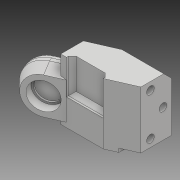
# Autodesk Inventor part: thumb_03 CMC top hinge
Saved by Autodesk Inventor 2017 SP1 (Build 210196100, 196)
## iProperties
Created: 2018-02-02
Part Number: thumb_03 CMC top hinge
Material: Generic
Document SubType Name: Modeling
Designer: JT
Density: 1 g/cm^3
Appearance: Default
Author: JT
Autodesk Inventor part; units mm, degrees
ref_plane "YZ Plane" through (0, 0, 0) normal (1, 0, 0) x (0, 1, 0)
sketch "Sketch1" plane through (0, 0, 0) normal (0, 0, 1) x (1, 0, 0)
  line L0 (0, 0) -> (-18, 0) construction
  line L1 (-9.705, 0) -> (-20.7027, -4.8012) construction
  line L2 (-20.7027, -4.8012) -> (-21.1028, -3.8847) construction
  dimension "d0" = 18
  dimension "d1" = 9.705
  dimension "d2" = 23.584
  dimension "d3" = 1
  dimension "d4" = 12
  constraints: 6 end point, 1 horizontal, 1 perpendicular, 1 point on line
  measures "d0" distance of L0.start L0.end
  measures "d1" distance of L0.start L1.start
  measures "d2" angle of L0 L1
  measures "d3" distance of L1.end L2.end
  measures "d4" distance of L1.start L1.end
ref_plane "Work Plane1" through (-20.7027, -4.8012, 0) normal (-0.4001, 0.9165, 0) x (-0.9165, -0.4001, 0)
sketch "Sketch3" plane through (-20.7027, -4.8012, 0) normal (-0.4001, 0.9165, 0) x (-0.9165, -0.4001, 0)
  circle A0 centre (0, 0) radius 6
  line L0 (0, -6) -> (-8, -6)
  line L1 (-8, -6) -> (-8, 6)
  line L2 (-8, 6) -> (0, 6)
  line L3 (0, 6) -> (0, -6)
  point P0 (-20.8944, 0)
  point P1 (0, 0)
  dimension "d8" = 12
  dimension "d13" = 8
  constraints: 8 end point, 3 horizontal, 2 parallel, 1 coincident, 1 perpendicular, 1 vertical alignment, 2 other
  measures "d13" distance from line of point (0, 0) L1
extrude "Extrusion2" add sketch "Sketch3" along normal blind 6
chamfer "Chamfer2" distance 3 angle 22 3 edges at (-26.2015, -7.2018, 0) (-17.0368, -3.2008, -6) (-17.0368, -3.2008, 6) measured on face at (-26.265, -5.0472, -3) measured on face at (-16.615, -0.8344, 6) measured on face at (-19.0589, -1.9013, -6)
sketch "Sketch2" plane through (0, 0, 0) normal (0, 0, 1) x (1, 0, 0)
  line L0 (-6.8718, -3) -> (-18, -3)
  line L1 (-18, -3) -> (-18, 2.9255)
  line L2 (-18, 2.9255) -> (0, 10.7837)
  line L3 (0, 10.7837) -> (0, 0)
  line L4 (-9.705, 0) -> (-20.7027, -4.8012) construction
  line L5 (-6.8718, -3) -> (0, 0)
  point P0 (0, 0)
  point P1 (-18, 0)
  point P2 (0, 0)
  dimension "d12" = 3
  dimension "d22" = 3
  dimension "d38" = 6
  constraints: 10 end point, 2 parallel, 2 point on line, 2 vertical, 1 horizontal
  measures "d12" distance from line of point (0, 0) L0
  measures "d22" distance from line of L0 L3.end
  measures "d38" distance between parallel lines of L2 L4
extrude "Extrusion1" add sketch "Sketch2" along normal blind 10 and the other way blind 6
sketch "Sketch5" plane through (-20.7027, -4.8012, 0) normal (0.4001, -0.9165, 0) x (0.9165, 0.4001, 0)
  point P0 (20.8944, 0)
  point P1 (0, 0)
hole "CMC bearing" at (-20.7027, -4.8012, 0) direction (-0.4001, 0.9165, 0) diameter 6 depth 3 counterbore diameter 7 counterbore depth 2.5
sketch "Sketch6" plane through (-18, -3, 10) normal (-1, 0, 0) x (0, 0, 1)
  line L0 (0, 5.9255) -> (0, 0) projected
  line L1 (0, 5.9255) -> (-4, 5.9255) projected
  line L2 (0, 0) -> (-4.982, 0) projected
  line L3 (-2, 5.9255) -> (-2, 0) construction
  point P0 (-10, 3)
  point P1 (-2, 2.9628)
  constraints: 2 end point, 2 midpoint, 1 perpendicular, 1 point on line
hole "top mount" at (-18, -0.0372, 8) direction (1, 0, 0) diameter 2 depth 8.5
sketch "Sketch8" plane through (-6.8718, -3, -6) normal (0, 0, -1) x (-1, 0, 0)
  line L0 (-6.8718, 3) -> (0, 0) projected
  line L1 (-6.8718, 13.7837) -> (-6.8718, 3) projected
  line L2 (16.2314, 3.6976) -> (-6.8718, 13.7837) projected
  line L3 (-2.8718, 1.2537) -> (-2.8718, 12.0374)
  dimension "d56" = 4
  constraints: 2 end point, 2 point on line, 1 vertical
  measures "d56" distance between parallel lines of L1 L3
extrude "Extrusion3" cut sketch "Sketch8" against normal blind 1
sketch "Sketch7" plane through (0, 0, 10) normal (1, 0, 0) x (0, 0, -1)
  line L0 (0, 10.7837) -> (15, 10.7837) projected
  line L1 (0, 0) -> (0, 10.7837) projected
  line L2 (0, 0) -> (15, 0) projected
  line L3 (7.5, 0) -> (7.5, 10.7837) construction
  line L4 (15, 0) -> (15, 10.7837) projected
  point P0 (10, 0)
  point P1 (2, 2.5)
  point P2 (13, 2.5)
  point P3 (7.5, 5.7837)
  dimension "d46" = 5
  dimension "d47" = 11
  dimension "d48" = 2.5
  constraints: 2 end point, 2 midpoint, 1 point on line, 1 symmetric about line
  measures "d46" distance from line of L0 point (7.5, 5.784)
  measures "d47" distance of point (13, 2.5) point (2, 2.5)
  measures "d48" distance from line of point (2, 2.5) L2
hole "bottom mount" at (0, 2.5, 8) at (0, 5.7837, 2.5) at (0, 2.5, -3) direction (-1, 0, 0) diameter 2 depth 8.5
sketch "Sketch9" plane through (-18, -3, -6) normal (0, -1, 0) x (1, 0, 0)
  line L0 (0, 16) -> (11.1282, 16) projected
  line L1 (11.1282, 16) -> (1.5, 16)
  line L2 (1.5, 16) -> (1.5, 7)
  line L3 (1.5, 7) -> (11.1282, 7)
  line L4 (11.1282, 7) -> (11.1282, 16)
  point P0 (18, 6)
  dimension "d59" = 9
  dimension "d60" = 1.5
  constraints: 8 end point, 2 parallel, 1 horizontal, 1 perpendicular
  measures "d59" distance between parallel lines of L0 L3
  measures "d60" distance from line of L2 L0.start
extrude "Extrusion4" cut sketch "Sketch9" against normal blind 1.5
chamfer "Chamfer3" distance 1 angle 45 3 edges at (-16.5, -1.5, 5.5) (-6.8718, -1.5, 5.5) (-11.6859, -1.5, 1)
ref_plane "Work Plane2" through (0, 8, 0) normal (0, 1, 0) x (-1, 0, 0)
split "Split1" plane through (0, 8, 0) removes the side toward (0, 1, 0)
chamfer "Chamfer4" distance 2 angle 45 1 edges at (-3.1882, 8, 10)
fillet "Fillet1" radius 2 3 edges at (-20.5516, 1.8116, 6) (-14.7398, 4.3488, -6) (-28.6021, -1.7029, 0)
equation "\"d2\" = thumb_axis_beta_local"
equation "\"thumb_axis_beta_local\" = thumb_axis_beta"
body "Solid1"
